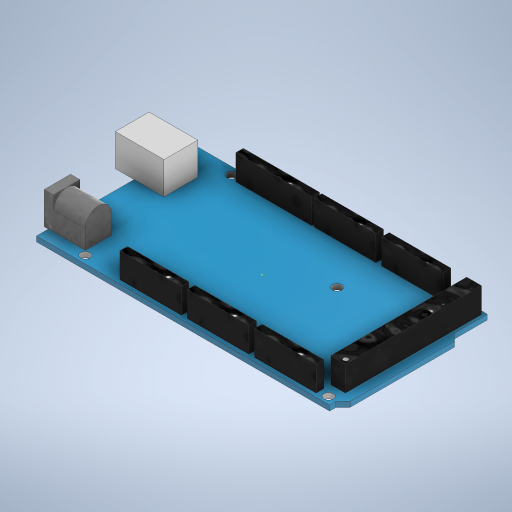
# Autodesk Inventor part: Arduino
Saved by Autodesk Inventor 2023 (Build 270158000, 158)
## iProperties
Created: 2023-09-14
Part Number: Arduino
Material: Generic
Document SubType Name: Modeling
Designer: Gage
Density: 1 g/cm^3
Appearance: Default
Author: Gage
Autodesk Inventor part; units mm, degrees
ref_plane "YZ Plane" through (0, 0, 0) normal (1, 0, 0) x (0, 1, 0)
ref_plane "XZ Plane" through (0, 0, 0) normal (0, 1, 0) x (-1, 0, 0)
ref_plane "XY Plane" through (0, 0, 0) normal (0, 0, 1) x (1, 0, 0)
sketch "Sketch1" plane through (0, 0, 0) normal (0, 1, 0) x (-1, 0, 0)
  line L0 (49.6094, -26.67) -> (-49.6094, -26.67)
  line L1 (-49.6094, -26.67) -> (-49.6094, 26.67)
  line L2 (-49.6094, 26.67) -> (49.6094, 26.67)
  line L3 (49.6094, 26.67) -> (49.6094, -26.67)
  line L4 (-51.9906, 22.1059) -> (-51.9906, -13.2159)
  line L5 (-51.9906, 22.1059) -> (-49.6094, 24.5323)
  line L6 (-51.9906, -13.2159) -> (-49.6094, -15.5529)
  point P0 (0, 0)
  point P1 (-49.6094, 0)
  point P2 (0, 26.67)
  dimension "d0" = 99.2188
  dimension "d1" = 53.34
  dimension "d2" = 101.6
  dimension "d3" = 35.3219
  dimension "d4" = 4.5641
  constraints: 14 end point, 2 midpoint, 2 parallel, 2 perpendicular, 2 point on line, 1 horizontal, 1 horizontal alignment, 1 vertical, 1 vertical alignment
  measures "d0" distance of L1.end L2.end
  measures "d1" distance of L0.end L1.end
  measures "d2" distance between parallel lines of L4 L3
  measures "d3" distance of L4.start L4.end
  measures "d4" vertical distance of L4.start L1.end
extrude "Extrusion1" add sketch "Sketch1" along normal blind 1.7859
sketch "Sketch2" plane through (0, 1.7859, 0) normal (0, 1, 0) x (1, 0, 0)
  point P0 (0, 0)
sketch "Sketch3" plane through (0, 1.7859, 0) normal (0, 1, 0) x (1, 0, 0)
  line L0 (23.0188, -22.8997) -> (43.8547, -22.8997)
  line L1 (43.8547, -22.8997) -> (43.8547, -25.4794)
  line L2 (43.8547, -25.4794) -> (23.0188, -25.4794)
  line L3 (23.0188, -25.4794) -> (23.0188, -22.8997)
  line L4 (-49.6094, -26.67) -> (49.6094, -26.67) projected
  line L5 (49.6094, -26.67) -> (49.6094, -24.5323) projected
  line L6 (0.1984, -22.8965) -> (21.0344, -22.8965)
  line L7 (21.0344, -22.8965) -> (21.0344, -25.4762)
  line L8 (21.0344, -25.4762) -> (0.1984, -25.4762)
  line L9 (0.1984, -25.4762) -> (0.1984, -22.8965)
  line L10 (-22.6219, -22.8965) -> (-1.7859, -22.8965)
  line L11 (-1.7859, -22.8965) -> (-1.7859, -25.4762)
  line L12 (-1.7859, -25.4762) -> (-22.6219, -25.4762)
  line L13 (-22.6219, -25.4762) -> (-22.6219, -22.8965)
  line L14 (17.6609, 25.4762) -> (38.4969, 25.4762)
  line L15 (38.4969, 25.4762) -> (38.4969, 22.8965)
  line L16 (38.4969, 22.8965) -> (17.6609, 22.8965)
  line L17 (17.6609, 22.8965) -> (17.6609, 25.4762)
  line L18 (49.6094, 15.5529) -> (49.6094, 26.67) projected
  line L19 (-5.1594, 25.4762) -> (15.6766, 25.4762)
  line L20 (15.6766, 25.4762) -> (15.6766, 22.8965)
  line L21 (15.6766, 22.8965) -> (-5.1594, 22.8965)
  line L22 (-5.1594, 22.8965) -> (-5.1594, 25.4762)
  line L23 (49.6094, 26.67) -> (-49.6094, 26.67) projected
  line L24 (-31.75, 25.4762) -> (-5.9531, 25.4762)
  line L25 (-5.9531, 25.4762) -> (-5.9531, 22.8965)
  line L26 (-5.9531, 22.8965) -> (-31.75, 22.8965)
  line L27 (-31.75, 22.8965) -> (-31.75, 25.4762)
  line L28 (43.8547, 25.5191) -> (48.8156, 25.5191)
  line L29 (48.8156, 25.5191) -> (48.8156, -20.5184)
  line L30 (48.8156, -20.5184) -> (43.8547, -20.5184)
  line L31 (43.8547, -20.5184) -> (43.8547, 25.5191)
  point P0 (0, 0)
  point P1 (49.6094, -25.6012)
  point P2 (43.8547, -24.1895)
  point P3 (21.0344, -24.1864)
  point P4 (-1.7859, -24.1864)
  point P5 (38.4969, 24.1864)
  point P6 (15.6766, 24.1864)
  dimension "d7" = 20.8359
  dimension "d8" = 2.5797
  dimension "d9" = 1.1906
  dimension "d10" = 5.7547
  dimension "d11" = 20.8359
  dimension "d12" = 2.5797
  dimension "d13" = 1.9844
  dimension "d14" = 1.1938
  dimension "d15" = 20.8359
  dimension "d16" = 2.5797
  dimension "d17" = 1.9844
  dimension "d18" = 1.1938
  dimension "d19" = 20.8359
  dimension "d20" = 2.5797
  dimension "d21" = 11.1125
  dimension "d22" = 20.8359
  dimension "d23" = 2.5797
  dimension "d24" = 1.9844
  dimension "d25" = 1.1938
  dimension "d26" = 1.1938
  dimension "d27" = 25.7969
  dimension "d28" = 2.5797
  dimension "d29" = 0.7937
  dimension "d30" = 1.1938
  dimension "d31" = 4.9609
  dimension "d32" = 46.0375
  dimension "d34" = 6.1516
  constraints: 56 end point, 8 parallel, 6 midpoint, 3 horizontal, 3 perpendicular
  measures "d7" distance of L1.end L2.end
  measures "d8" distance of L0.end L1.end
  measures "d9" distance between parallel lines of L4 L2
  measures "d10" horizontal distance of point (49.609, -25.601) point (43.855, -24.19)
  measures "d11" distance of L7.end L8.end
  measures "d12" distance of L6.end L7.end
  measures "d13" distance between parallel lines of L3 L7
  measures "d14" distance between parallel lines of L8 L4
  measures "d15" distance of L11.end L12.end
  measures "d16" distance of L10.end L11.end
  measures "d17" distance between parallel lines of L9 L11
  measures "d18" distance between parallel lines of L4 L12
  measures "d19" distance of L15.end L16.end
  measures "d20" distance of L14.end L15.end
  measures "d21" distance between parallel lines of L18 L15
  measures "d22" distance of L21.start L22.start
  measures "d23" distance of L19.end L21.start
  measures "d24" distance between parallel lines of L17 L20
  measures "d25" distance between parallel lines of L23 L14
  measures "d26" distance between parallel lines of L23 L19
  measures "d27" distance of L25.end L26.end
  measures "d28" distance of L24.end L25.end
  measures "d29" distance between parallel lines of L22 L25
  measures "d30" distance between parallel lines of L23 L24
  measures "d31" distance of L29.end L30.end
  measures "d32" distance of L28.end L29.end
  measures "d34" distance between parallel lines of L4 L30
extrude "Extrusion2" add sketch "Sketch3" along normal blind 8.5328
sketch "Sketch4" plane through (0, 1.7859, 0) normal (0, 1, 0) x (1, 0, 0)
  line L0 (-50.9984, -13.7716) -> (-37.1078, -13.7716)
  line L1 (-37.1078, -13.7716) -> (-37.1078, -22.7013)
  line L2 (-37.1078, -22.7013) -> (-50.9984, -22.7013)
  line L3 (-50.9984, -22.7013) -> (-50.9984, -13.7716)
  line L4 (-49.6094, 26.67) -> (-49.6094, -26.67) projected
  line L5 (-49.6094, -26.67) -> (49.6094, -26.67) projected
  point P0 (0, 0)
  point P1 (-50.9984, -18.2364)
  point P2 (-49.6094, -13.7716)
  point P3 (-49.6094, -22.7013)
  dimension "d37" = 13.8906
  dimension "d38" = 8.9297
  dimension "d39" = 1.3891
  dimension "d40" = 3.9688
  constraints: 8 end point, 2 parallel, 1 horizontal, 1 midpoint, 1 perpendicular
  measures "d37" distance of L1.end L2.end
  measures "d38" distance of L0.end L1.end
  measures "d39" distance from line of point (-50.998, -18.236) L4
  measures "d40" distance between parallel lines of L2 L5
extrude "Extrusion3" add sketch "Sketch4" along normal blind 10.9141
sketch "Sketch5" plane through (-37.1078, 1.7859, 22.7013) normal (1, 0, 0) x (0, 0, -1)
  circle A0 centre (4.4648, 6.4437) radius 4.4648
  line L0 (0, 0) -> (0, 10.9141) projected
  line L1 (0, 10.9141) -> (8.9297, 10.9141) projected
  line L2 (8.9297, 10.9141) -> (0, 10.9141) projected
  line L3 (4.4648, 10.9141) -> (0, 10.9141)
  line L4 (0, 10.9141) -> (0, 6.4437)
  line L5 (0, 0) -> (0, 10.9141) projected
  line L6 (8.9297, 0) -> (8.9297, 10.9141) projected
  line L7 (8.9297, 6.4437) -> (8.9297, 10.9141)
  line L8 (8.9297, 10.9141) -> (4.4648, 10.9141)
  point P0 (22.7013, -1.7859)
  point P1 (0, 6.4437)
  dimension "d44" = 8.9297
  dimension "d45" = 4.4648
  dimension "d46" = 4.4704
  constraints: 8 end point, 2 collinear, 2 point on circle, 2 point on line, 1 centre point, 1 midpoint, 1 perpendicular
  measures "d44" diameter of A0
  measures "d45" distance from line of L0 A0.centre
  measures "d46" distance from line of A0.centre L1
extrude "Extrusion4" cut sketch "Sketch5" against normal blind 10.7156 contours A0 L0 L1 L6
sketch "Sketch6" plane through (0, 1.7859, 0) normal (0, 1, 0) x (1, 0, 0)
  line L0 (-55.9594, 17.78) -> (-39.4938, 17.78)
  line L1 (-39.4938, 17.78) -> (-39.4938, 6.35)
  line L2 (-39.4938, 6.35) -> (-55.9594, 6.35)
  line L3 (-55.9594, 6.35) -> (-55.9594, 17.78)
  line L4 (49.6094, 26.67) -> (-49.6094, 26.67) projected
  line L5 (-49.6094, 26.67) -> (-49.6094, -13.7716) projected
  point P0 (0, 0)
  point P1 (-49.6094, -13.7914)
  dimension "d49" = 16.4656
  dimension "d50" = 11.43
  dimension "d51" = 8.89
  dimension "d52" = 6.35
  constraints: 8 end point, 2 parallel, 1 horizontal, 1 perpendicular
  measures "d49" distance of L1.end L2.end
  measures "d50" distance of L0.end L1.end
  measures "d51" distance between parallel lines of L4 L0
  measures "d52" distance between parallel lines of L5 L3
extrude "Extrusion5" add sketch "Sketch6" along normal blind 10.9141
sketch "Sketch7" plane through (0, 1.7859, 0) normal (0, 1, 0) x (1, 0, 0)
  circle A0 centre (-34.3694, 24.13) radius 1.5875
  line L0 (-49.6094, 26.67) -> (-49.6094, 17.78) projected
  line L1 (49.6094, 26.67) -> (-49.6094, 26.67) projected
  circle A1 centre (-35.6394, -24.13) radius 1.5875
  line L2 (-49.6094, -26.67) -> (49.6094, -26.67) projected
  circle A2 centre (40.5606, 24.2888) radius 1.5875
  circle A3 centre (46.9106, -24.3086) radius 1.5875
  line L3 (-49.6094, 26.67) -> (-49.6094, -26.67) projected
  circle A4 centre (16.4306, 9.0488) radius 1.5875
  circle A5 centre (16.4306, -18.8913) radius 1.5875
  point P0 (0, 0)
  point P1 (-49.6094, -22.7211)
  point P2 (-49.6094, 0)
  point P3 (-49.6094, 0)
  dimension "d55" = 3.175
  dimension "d56" = 15.24
  dimension "d57" = 2.54
  dimension "d58" = 3.175
  dimension "d59" = 2.54
  dimension "d60" = 3.175
  dimension "d62" = 2.3813
  dimension "d63" = 3.175
  dimension "d65" = 13.97
  dimension "d66" = 3.175
  dimension "d67" = 50.8
  dimension "d68" = 17.6212
  dimension "d69" = 3.175
  dimension "d70" = 27.94
  dimension "d78" = 96.52
  dimension "d79" = 90.17
  constraints: 6 centre point, 2 midpoint
  measures "d55" diameter of A0
  measures "d56" distance from line of A0.centre L0
  measures "d57" distance from line of L1 A0.centre
  measures "d58" diameter of A1
  measures "d59" distance from line of L2 A1.centre
  measures "d60" diameter of A2
  measures "d62" distance from line of L1 A2.centre
  measures "d63" diameter of A3
  measures "d65" horizontal distance of point (-49.609, 0) A1.centre
  measures "d66" diameter of A4
  measures "d67" horizontal distance of A4.centre A0.centre
  measures "d68" distance from line of L1 A4.centre
  measures "d69" diameter of A5
  measures "d70" distance of A5.centre A4.centre
  measures "d78" horizontal distance of A3.centre point (-49.609, 0)
  measures "d79" distance from line of A2.centre L0
hole "Hole1" at (-35.6394, 1.7859, 24.13) at (16.4306, 1.7859, -9.0488) at (40.5606, 1.7859, -24.2888) at (46.9106, 1.7859, 24.3086) at (-34.3694, 1.7859, -24.13) at (16.4306, 1.7859, 18.8913) direction (0, -1, 0) diameter 3.175 end through all start extended yes
sketch "Sketch8" plane through (-55.9594, 1.7859, -17.78) normal (-1, 0, 0) x (0, 0, 1)
  line L0 (0.9525, 1.6071) -> (10.4775, 1.6071)
  line L1 (11.43, 0) -> (11.43, 10.9141) projected
  line L2 (10.4775, 1.6071) -> (10.4775, 6.3823)
  line L3 (10.4775, 6.3823) -> (10.4775, 6.3823)
  line L4 (10.4775, 6.3823) -> (7.3344, 9.5254)
  line L5 (0.9525, 1.6071) -> (0.9525, 6.3823)
  line L6 (0, 0) -> (0, 10.9141) projected
  line L7 (0.9525, 1.6071) -> (5.7277, 1.6071) construction
  line L8 (38.2984, 8.5328) -> (-7.7391, 8.5328) projected
  line L9 (0.9525, 6.3823) -> (4.0956, 9.5254)
  line L10 (0.9525, 6.3823) -> (5.3975, 6.3823) construction
  line L11 (4.0956, 9.5254) -> (7.3344, 9.5254)
  line L12 (0, 0) -> (11.43, 0) projected
  line L13 (4.0956, 6.8519) -> (7.3344, 6.8519)
  line L14 (7.3344, 6.8519) -> (7.3344, 3.1435)
  line L15 (7.3344, 3.1435) -> (4.0956, 3.1435)
  line L16 (4.0956, 3.1435) -> (4.0956, 6.8519)
  point P0 (17.78, -1.7859)
  point P1 (5.715, 1.6071)
  point P2 (5.715, 0)
  dimension "d81" = 4.7752
  dimension "d82" = 90
  dimension "d83" = 9.525
  dimension "d84" = 4.7752
  dimension "d85" = 90
  dimension "d86" = 4.445
  dimension "d87" = 135
  dimension "d89" = 4.445
  dimension "d90" = 45
  dimension "d91" = 90
  constraints: 26 end point, 4 horizontal, 3 parallel, 2 equal length, 2 midpoint, 1 perpendicular, 1 point on line, 1 vertical, 1 vertical alignment
  measures "d81" distance of L0.start L5.end
  measures "d82" angle of L7 L5
  measures "d83" distance of L0.start L0.end
  measures "d84" distance of L0.end L2.end
  measures "d85" angle of L0 L2
  measures "d86" distance of L3.end L4.end
  measures "d87" angle of L2 L4
  measures "d89" distance of L5.end L9.end
  measures "d90" angle of L10 L9
  measures "d91" angle of L5 L10
extrude "Extrusion6" cut sketch "Sketch8" against normal blind 6.35 contours L5 L9 L8 L4 L2 L0 | L9 L11 L4 L8
sketch "Sketch9" plane through (-50.9984, 1.7859, 13.7716) normal (-1, 0, 0) x (0, 0, 1)
  circle A0 centre (4.4847, 6.35) radius 3.175
  circle A1 centre (4.4847, 6.35) radius 1.5875
  line L0 (8.9297, 0) -> (8.9297, 10.9141) projected
  point P0 (-13.7716, -1.7859)
  dimension "d94" = 3.175
  dimension "d95" = 4.445
  constraints: 2 centre point, 1 coincident
  measures "d94" diameter of A1
  measures "d95" distance from line of L0 A0.centre
extrude "Extrusion7" cut sketch "Sketch9" against normal blind 6.35
sketch "Sketch10" plane through (0, 10.3187, 0) normal (0, 1, 0) x (1, 0, 0)
  circle A0 centre (47.4694, -19.05) radius 0.8001
  line L0 (48.8156, -20.5184) -> (48.8156, 25.5191) projected
  line L1 (43.8547, 25.5191) -> (43.8547, -20.5184) projected
  point P0 (0, 0)
  point P1 (47.625, -7.9375)
  point P2 (45.2009, -19.05)
  dimension "d98" = 1.6002
  dimension "d101" = 1.3462
  dimension "d102" = 1.3462
  constraints: 1 centre point
  measures "d98" diameter of A0
  measures "d101" distance from line of L0 A0.centre
  measures "d102" distance from line of L1 point (45.201, -19.05)
extrude "Extrusion8" cut sketch "Sketch10" against normal blind 2.54
body "Solid1"
